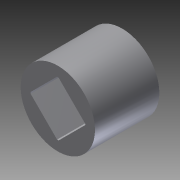
# Autodesk Inventor part: Поз5 Муфта
Saved by Autodesk Inventor 2012 SP2 (Build 160219200, 219)
## iProperties
Created: 2014-03-31
Part Number: Поз5 Муфта
Material: Default
Document SubType Name: Modeling
Designer: Student
Density: 1 g/cm^3
Mass: 1.46658 g
Surface Area: 12.4788 cm^2
Volume: 1.46658 cm^3
Author: Student
Autodesk Inventor part; units mm, degrees
ref_plane "YZ Plane" through (0, 0, 0) normal (1, 0, 0) x (0, 1, 0)
ref_plane "XZ Plane" through (0, 0, 0) normal (0, 1, 0) x (-1, 0, 0)
ref_plane "XY Plane" through (0, 0, 0) normal (0, 0, 1) x (1, 0, 0)
sketch "Эскиз1" plane through (0, 0, 0) normal (0, 1, 0) x (-1, 0, 0)
  line L0 (-0.1311, -5.5) -> (-5.5, -0.1311)
  line L1 (-5.5, 0.1311) -> (-0.1311, 5.5)
  line L2 (0.1311, 5.5) -> (5.5001, 0.131)
  line L3 (5.5001, -0.131) -> (0.1311, -5.5)
  line L4 (-5.5, 0.131) -> (-5.5, -0.1311)
  line L5 (5.5001, 0.131) -> (5.5001, -0.131)
  line L6 (-0.131, 5.5) -> (0.1311, 5.5)
  line L7 (0.1311, -5.5) -> (-0.1311, -5.5)
  circle A0 centre (0, 0) radius 7.5
  constraints: 16 end point, 2 parallel, 2 point on line, 1 centre point, 1 coincident, 1 perpendicular, 1 vertical, 5 other
extrude "Выдавливание1" add sketch "Эскиз1" along normal blind 13 contours L0 L4 L1 L6 L2 L5 L3 L7 | A0
sketch "Эскиз2" plane through (0, 0, 0) normal (0, -1, 0) x (1, 0, 0)
  circle A0 centre (0, 0) radius 7.5 projected
  line L0 (0.1555, 5.5004) -> (5.5383, 0.1184)
  line L1 (5.5386, -0.1173) -> (0.1571, -5.4996)
  line L2 (-0.156, -5.4999) -> (-5.4995, -0.1573)
  line L3 (-5.4998, 0.1561) -> (-0.0021, 5.6547)
  line L4 (5.5383, 0.1184) -> (5.5386, -0.1173)
  line L5 (-5.4995, -0.1573) -> (-5.4998, 0.1561)
  line L6 (0.1555, 5.5004) -> (-0.1567, 5.5001)
  line L7 (-0.156, -5.4999) -> (0.1571, -5.4996)
  dimension "d4" = 8
  dimension "d5" = 11
  constraints: 16 end point, 2 parallel, 1 coincident, 1 perpendicular, 1 point on line, 5 other
  measures "d4" distance of L2.end L3.end
  measures "d5" distance of L0.start L1.end
extrude "Выдавливание2" cut sketch "Эскиз2" against normal blind 13 contours L0 L4 L1 L7 L2 L5 L3 L6
